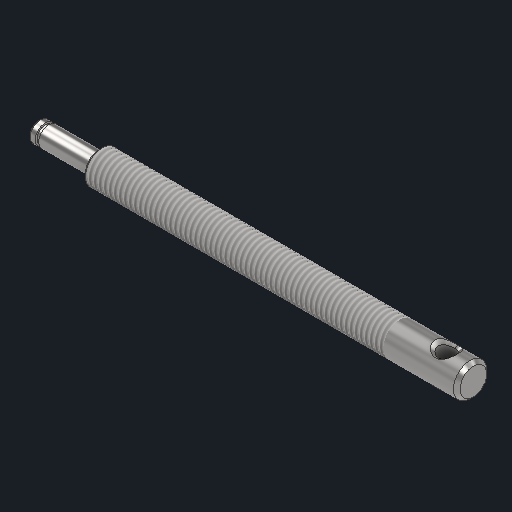
# Autodesk Inventor part: Rod
Saved by Autodesk Inventor 2025.4 (Build 294407000, 407)
## iProperties
Created: 2026-05-27
Part Number: Rod
Material: Stainless Steel
Document SubType Name: Modeling
Designer: VuQuan
Density: 8 g/cm^3
Appearance: Semi-Polished
Author: VuQuan
Autodesk Inventor part; units mm, degrees
ref_plane "YZ Plane" through (0, 0, 0) normal (1, 0, 0) x (0, 1, 0)
ref_plane "XZ Plane" through (0, 0, 0) normal (0, 1, 0) x (-1, 0, 0)
ref_plane "XY Plane" through (0, 0, 0) normal (0, 0, 1) x (1, 0, 0)
sketch "Sketch1" plane through (0, 0, 0) normal (0, 0, 1) x (1, 0, 0)
  line L0 (0, 0) -> (0, 3)
  line L1 (0, 3) -> (2, 3)
  line L2 (2, 3) -> (2, 2.5)
  line L3 (2, 2.5) -> (3, 2.5)
  line L4 (3, 2.5) -> (3, 3)
  line L5 (3, 3) -> (18, 3)
  line L6 (18, 3) -> (18, 5)
  line L7 (18, 5) -> (130, 5)
  line L8 (130, 5) -> (130, 0)
  line L9 (130, 0) -> (0, 0)
  line L10 (122, 5) -> (122, 0)
  dimension "d0" = 1
  dimension "d2" = 3
  dimension "d3" = 6
  dimension "d4" = 5
  dimension "d5" = 130
  dimension "d6" = 18
  dimension "d7" = 10
  dimension "d8" = 8
  constraints: 22 end point, 6 perpendicular, 3 point on line, 2 parallel, 1 horizontal, 1 vertical
  measures "d0" distance of L2.end L3.end
  measures "d2" distance between parallel lines of L0 L4
  measures "d3" diameter of L1 L9
  measures "d4" diameter of L3 L9
  measures "d5" distance between parallel lines of L8 L0
  measures "d6" distance between parallel lines of L6 L0
  measures "d7" diameter of L7 L9
  measures "d8" distance between parallel lines of L8 L10
revolve "Revolution1" add sketch "Sketch1" angle 360 about axis through (130, 0, 0) along (-1, 0, 0)
thread "Thread1" size "M10x1.5" class "6g" standard "ISO Metric profile" length 90
chamfer "Chamfer2" distance 0.5 angle 45 1 edges at (0, -3, 0)
sketch "Sketch2" plane through (0, 0, 0) normal (0, 1, 0) x (-1, 0, 0)
  circle A0 centre (-122, 0) radius 2.5
  point P0 (0, 0)
  dimension "d21" = 5
  constraints: 1 centre point, 1 coincident
  measures "d21" diameter of A0
extrude "Extrusion1" cut sketch "Sketch2" along normal through all both and the other way through all
chamfer "Chamfer3" distance 1 angle 45 5 edges at (18, -5, 0) (130, -5, 0) (121.9995, 4.3301, -2.5) (122.0005, 4.3301, 2.5) (124.4999, -5, -0.0199)
body "Solid1"
